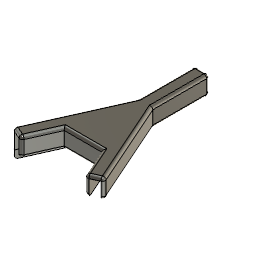
Drop Ceiling_Middle Connector_Right (Autodesk Fusion 360 design; units mm, degrees)
Autodesk Fusion 360 part; units mm, degrees
sketch "Base MC 1" plane through (0, 0, 0) normal (0, 0, 1) x (1, 0, 0)
  line L0 (-8.2378, 52.2598) -> (7.2122, 52.2598)
  line L1 (-8.2378, 52.2598) -> (-8.2378, -7.7402)
  line L2 (7.2122, 52.2598) -> (7.2122, -7.7402)
  line L3 (-8.2378, -7.7402) -> (-48.9115, -99.0948)
  line L4 (-8.2378, -7.7402) -> (94.6998, -7.7402) construction
  line L5 (7.2122, -7.7402) -> (47.8859, -99.0948)
  line L6 (7.2122, -7.7402) -> (110.1498, -7.7402) construction
  line L7 (-20.5128, -73.2956) -> (19.4872, -73.2956)
  line L8 (-48.9115, -99.0948) -> (-34.7972, -105.3789)
  line L9 (47.8859, -99.0948) -> (33.7716, -105.3789)
  line L10 (-34.7972, -105.3789) -> (-20.5128, -73.2956)
  line L11 (33.7716, -105.3789) -> (19.4872, -73.2956)
  dimension "d1" = 15.45
  dimension "d2" = 60
  dimension "d3" = 60
  dimension "d4" = 114
  dimension "d5" = 100
  dimension "d6" = 66
  dimension "d7" = 100
  dimension "d8" = 40
  dimension "d9" = 15.45
  dimension "d10" = 15.45
  constraint horizontal L0
  constraint perpendicular L0 L1
  constraint perpendicular L0 L2
  constraint horizontal L4
  constraint coincident L1 L3.start
  constraint horizontal L6
  constraint coincident L4 L2.end
  constraint coincident L2 L5.start
  constraint horizontal L7
  constraint perpendicular L3 L8
  constraint perpendicular L5 L9
  constraint perpendicular L8 L10
  constraint perpendicular L9 L11
  measures "d1" distance of L0.start L0.end
  measures "d2" distance of L0.start L1.end
  measures "d3" distance of L0.end L2.end
  measures "d4" angle of L3 L4
  measures "d5" distance of L1.end L3.end
  measures "d6" angle of L5 L6
  measures "d7" distance of L2.end L5.end
  measures "d8" distance of L7.start L7.end
  measures "d9" distance of L3.end L8.end
  measures "d10" distance of L5.end L9.end
extrude "Extrude1" add sketch "Base MC 1" along normal blind 20
sketch "Cut-Outs MC1" plane through (0, 0, 0) normal (0, 0, 1) x (1, 0, 0)
  line L0 (-5.2378, 52.2642) -> (4.2122, 52.2642)
  line L1 (-5.2378, 52.2642) -> (-5.2378, -17.7358)
  line L2 (4.2122, 52.2642) -> (4.2122, -17.7358)
  line L3 (4.2122, -17.7358) -> (-5.2378, -17.7358)
  line L4 (-8.2378, 52.2598) -> (-8.2378, -7.7402)
  line L5 (-37.5379, -104.1589) -> (-46.1709, -100.3152)
  line L6 (-37.5379, -104.1589) -> (-28.0879, -104.1589) construction
  line L7 (-46.1709, -100.3152) -> (-25.8341, -54.6379)
  line L8 (-37.5379, -104.1589) -> (-17.2011, -58.4816)
  line L9 (-25.8341, -54.6379) -> (-17.2011, -58.4816)
  line L10 (-34.7972, -105.3789) -> (-20.5128, -73.2956)
  line L11 (36.5123, -104.1589) -> (45.1453, -100.3152)
  line L12 (36.5123, -104.1589) -> (45.9621, -104.1589) construction
  line L13 (45.1453, -100.3152) -> (24.8085, -54.6379)
  line L14 (36.5123, -104.1589) -> (16.1755, -58.4816)
  line L15 (16.1755, -58.4816) -> (24.8085, -54.6379)
  line L16 (7.2122, -7.7402) -> (47.8859, -99.0948)
  dimension "d13" = 9.45
  dimension "d14" = 70
  dimension "d15" = 70
  dimension "d16" = 3
  dimension "d17" = 156
  dimension "d18" = 9.45
  dimension "d19" = 50
  dimension "d20" = 50
  dimension "d21" = 3
  dimension "d22" = 24
  dimension "d23" = 9.45
  dimension "d24" = 50
  dimension "d25" = 50
  dimension "d26" = 3
  constraint horizontal L0
  constraint perpendicular L0 L1
  constraint perpendicular L0 L2
  constraint horizontal L6
  constraint perpendicular L5 L7
  constraint perpendicular L5 L8
  constraint horizontal L12
  constraint perpendicular L11 L13
  constraint perpendicular L11 L14
  measures "d13" distance of L0.start L0.end
  measures "d14" distance of L0.start L1.end
  measures "d15" distance of L0.end L2.end
  measures "d16" distance of L1 L4
  measures "d17" angle of L5 L6
  measures "d18" distance of L5.start L5.end
  measures "d19" distance of L5.end L7.end
  measures "d20" distance of L5.start L8.end
  measures "d21" distance of L8 L10
  measures "d22" angle of L11 L12
  measures "d23" distance of L11.start L11.end
  measures "d24" distance of L11.end L13.end
  measures "d25" distance of L11.start L14.end
  measures "d26" distance of L13 L16
extrude "Extrude2" cut sketch "Cut-Outs MC1" along normal blind 17
sketch "Upper-Extend MC1" plane through (0, 0, 0) normal (0, 0, 1) x (1, 0, 0)
  line L0 (-46.1708, -100.315) -> (-5.2367, -8.3755)
  line L1 (-46.1708, -100.315) -> (54.4694, -100.315) construction
  line L2 (-5.2367, -8.3755) -> (-5.2367, 52.2617)
  line L3 (-5.2367, 52.2617) -> (-8.2367, 52.2617)
  line L4 (-8.2367, 52.2617) -> (-8.2367, -7.7379)
  line L5 (-8.2367, -7.7379) -> (-48.9121, -99.0963)
  line L6 (-48.9121, -99.0963) -> (-46.1708, -100.315)
  dimension "d29" = 66
  dimension "d30" = 3
  dimension "d31" = 3
  constraint horizontal L1
  constraint vertical L2
  constraint perpendicular L2 L3
  constraint perpendicular L3 L4
  constraint parallel L0 L5
  measures "d29" angle of L0 L1
  measures "d30" distance of L2 L4
  measures "d31" distance of L0 L5
extrude "Extrude3" add sketch "Upper-Extend MC1" against normal blind 8.5
fillet "Fillet4" radius 2.95 31 edges at (-8.2378, 22.2598, 20) (-28.5746, -53.4175, 20) (-41.8543, -102.2368, 20) (-27.655, -89.3372, 20) (-0.5128, -73.2956, 20) (26.6294, -89.3372, 20) (40.8287, -102.2368, 20) (27.549, -53.4175, 20) (7.2122, 22.2598, 20) (-0.5128, 52.2598, 20) (27.549, -53.4175, 0) (7.2122, 22.2598, 0) (-28.5744, -53.4171, -8.5) (-8.2367, 22.2619, -8.5) (-48.9115, -99.0948, 10) (-48.9121, -99.0963, -4.25) (-8.2378, 52.2598, 10) (-8.2367, 52.2617, -4.25) (7.2122, 52.2598, 10) (47.8859, -99.0948, 10) (-34.7972, -105.3789, 10) (-27.655, -89.3372, 0) (-0.5128, -73.2956, 0) (26.6294, -89.3372, 0) (-36.1675, -104.7688, 0) (35.1419, -104.7688, 0) (46.5156, -99.7049, 0) (-6.7367, 52.2617, -8.5) (5.7122, 52.2598, 0) (-47.5415, -99.7056, -8.5) (33.7716, -105.3789, 10)
equation "d1 = 9.45 mm + 3 mm + 3 mm"
equation "d3 = d2"
equation "d4 = 90 deg + 24 deg"
equation "d6 = 90 deg - 24 deg"
equation "d7 = d5"
equation "d9 = d1"
equation "d10 = d1"
equation "d15 = d14"
equation "d16 = ( d1 - d13 ) / 2"
equation "d20 = d19"
equation "d21 = ( d9 - d18 ) / 2"
equation "d25 = d24"
equation "d26 = ( d10 - d23 ) / 2"
equation "d30 = d16"
equation "d31 = d21"
named bodies: "Middle Connector V1"
